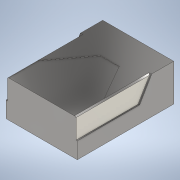
# Autodesk Inventor part: Port 1
Saved by Autodesk Inventor 2020 (Build 240168000, 168)
## iProperties
Created: 2022-11-24
Part Number: Port 1
Material: Generic
Document SubType Name: Modeling
Designer: DELL
Density: 1 g/cm^3
Appearance: Steel - Polished
Author: DELL
Autodesk Inventor part; units mm, degrees
ref_plane "YZ Plane" through (0, 0, 0) normal (1, 0, 0) x (0, 1, 0)
ref_plane "XZ Plane" through (0, 0, 0) normal (0, 1, 0) x (-1, 0, 0)
ref_plane "XY Plane" through (0, 0, 0) normal (0, 0, 1) x (1, 0, 0)
sketch "Sketch1" plane through (0, 0, 0) normal (0, 1, 0) x (-1, 0, 0)
  line L0 (0, 0) -> (0, 39)
  line L1 (0, 39) -> (-28.713, 39)
  line L2 (-28.713, 39) -> (-28.713, 0)
  line L3 (-28.713, 0) -> (0, 0)
  dimension "d0" = 39
  dimension "d1" = 28.713
  constraints: 8 end point, 3 perpendicular, 1 vertical
  measures "d0" distance of L0.start L0.end
  measures "d1" distance of L0.end L1.end
extrude "Extrusion1" add sketch "Sketch1" along normal blind 15
sketch "Sketch2" plane through (28.713, 0, 0) normal (0, 0, -1) x (-1, 0, 0)
  line L0 (28.713, 0) -> (28.713, 15) projected
  line L1 (0, 0) -> (28.713, 0) projected
  line L2 (2, 12) -> (26.713, 12)
  line L3 (2, 5.0411) -> (4.5, 5.0411)
  line L4 (4.5, 5.0411) -> (4.5, 2.0411)
  line L5 (4.5, 2.0411) -> (6, 2.0411)
  line L6 (6, 2.0411) -> (6, 0.5411)
  line L7 (6, 0.5411) -> (19.8539, 0.5411)
  line L8 (26.713, 5.0411) -> (24.213, 5.0411)
  line L9 (24.213, 5.0411) -> (24.213, 2.0411)
  line L10 (24.213, 2.0411) -> (22.713, 2.0411)
  line L11 (22.713, 2.0411) -> (22.713, 0.5411)
  line L12 (22.713, 0.5411) -> (19.8539, 0.5411)
  line L13 (2, 12) -> (2, 5.0411)
  line L14 (26.713, 12) -> (26.713, 5.0411)
  point P0 (0, 15)
  dimension "d7" = 2.5
  dimension "d8" = 3
  dimension "d9" = 1.5
  dimension "d10" = 1.5
  dimension "d11" = 2.5
  dimension "d12" = 3
  dimension "d13" = 1.5
  dimension "d14" = 1.5
  constraints: 26 end point, 6 perpendicular, 1 vertical
  measures "d7" distance of L3.start L3.end
  measures "d8" distance of L3.end L4.end
  measures "d9" distance of L4.end L5.end
  measures "d10" distance of L5.end L6.end
  measures "d11" distance of L8.start L8.end
  measures "d12" distance of L8.end L9.end
  measures "d13" distance of L9.end L10.end
  measures "d14" distance of L10.end L11.end
extrude "Extrusion2" cut sketch "Sketch2" against normal blind 35
sketch "Sketch3" plane through (28.713, 0, 39) normal (1, 0, 0) x (0, 0, -1)
  line L0 (25.0019, 6.616) -> (0, 6.616)
  line L1 (0, 0) -> (0, 15) projected
  line L2 (25.0019, 6.616) -> (29.9465, 15)
  line L3 (0, 15) -> (39, 15) projected
  line L4 (29.9465, 15) -> (0, 15)
  line L5 (0, 6.616) -> (0, 15)
  point P0 (39, 0)
  constraints: 8 end point, 2 perpendicular, 2 point on line, 1 horizontal
extrude "Extrusion3" cut sketch "Sketch3" against normal blind 0.5
chamfer "Chamfer1" distance 0.2 angle 45 1 edges at (28.713, 10.808, 11.5258)
sketch "Sketch4" plane through (0, 0, 0) normal (-1, 0, 0) x (0, 0, 1)
  line L0 (13.9981, 6.616) -> (39, 6.616) projected
  line L1 (39, 6.616) -> (13.9981, 6.616)
  line L2 (9.0535, 15) -> (13.9981, 6.616) projected
  line L3 (13.9981, 6.616) -> (9.0535, 15)
  line L4 (0, 15) -> (39, 15) projected
  line L5 (9.0535, 15) -> (39, 15)
  line L6 (39, 15) -> (39, 6.616)
  line L7 (39, 0) -> (39, 15) projected
  point P0 (0, 0)
  constraints: 8 end point, 4 collinear
extrude "Extrusion4" cut sketch "Sketch4" against normal blind 0.5
chamfer "Chamfer2" distance 0.5 angle 45 2 edges at (0.5, 15, 24.0267) (28.213, 15, 24.0267)
sketch "Sketch5" plane through (0, 15, 0) normal (0, 1, 0) x (1, 0, 0)
  line L0 (27.713, -9.0535) -> (27.713, -39) projected
  line L1 (27.713, -27.1604) -> (19.4998, -12.8142)
  line L2 (19.4998, -12.8142) -> (11.8392, -12.8142)
  line L3 (27.713, -39) -> (28.213, -39) projected
  line L4 (27.713, -27.1604) -> (27.713, -39)
  line L5 (1, -39) -> (27.713, -39) projected
  line L6 (27.713, -39) -> (1, -39)
  line L7 (1, -39) -> (1, -27.1604)
  line L8 (1, -39) -> (1, -9.0535) projected
  line L9 (1, -27.1604) -> (11.8392, -12.8142)
  point P0 (0, 0)
  constraints: 12 end point, 2 perpendicular, 2 point on line, 1 vertical
extrude "Extrusion5" cut sketch "Sketch5" against normal blind 0.2
body "Solid1"
